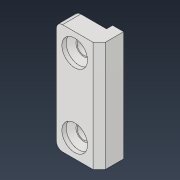
# Autodesk Inventor part: IR Schutz
Saved by Autodesk Inventor 2022.1 (Build 261234020, 234B)
## iProperties
Part Number: IR Schutz
Material: PC/ABS-Kunststoff
Document SubType Name: Modeling
Designer: rYan
Density: 0.357273 g/cm^3
Appearance: Glatt - weiß
Mass: 0.102481 g
Surface Area: 4.81339 cm^2
Volume: 0.286842 cm^3
Author: rYan
Autodesk Inventor part; units mm, degrees
ref_plane "YZ Plane" through (0, 0, 0) normal (1, 0, 0) x (0, 1, 0)
ref_plane "XZ Plane" through (0, 0, 0) normal (0, 1, 0) x (-1, 0, 0)
ref_plane "XY Plane" through (0, 0, 0) normal (0, 0, 1) x (1, 0, 0)
sketch "Skizze1" plane through (0, 0, 0) normal (0, 1, 0) x (-1, 0, 0)
  line L0 (3.5, -9) -> (-3.5, -9)
  line L1 (-3.5, -9) -> (-3.5, 9)
  line L2 (-3.5, 9) -> (3.5, 9)
  line L3 (3.5, 9) -> (3.5, -9)
  line L4 (3.5, -9) -> (-3.5, 9) construction
  line L5 (-3.5, -9) -> (3.5, 9) construction
  line L6 (0.5, 6) -> (0.5, -6) construction
  circle A0 centre (0.5, 6) radius 1.1
  circle A1 centre (0.5, -6) radius 1.1
  point P0 (0, 0)
  dimension "d0" = 7
  dimension "d1" = 18
  dimension "d2" = 2.2
  dimension "d4" = 12
  dimension "d5" = 3
  dimension "d6" = 4
  constraints: 14 end point, 2 centre point, 2 coincident, 2 midpoint, 2 parallel, 1 equal radius, 1 horizontal, 1 perpendicular, 1 vertical
  measures "d0" distance of L1.end L2.end
  measures "d1" distance of L0.end L1.end
  measures "d2" diameter of A0
  measures "d4" distance of L6.start L6.end
  measures "d5" distance from line of L0 L6.end
  measures "d6" distance from line of L1 L6.end
extrude "Extrusion1" add sketch "Skizze1" along normal blind 4
sketch "Skizze3" plane through (0, 4, 0) normal (0, 1, 0) x (1, 0, 0)
  circle A0 centre (-0.5, 6) radius 1.1 projected
  circle A1 centre (-0.5, -6) radius 1.1 projected
  line L0 (3.5, 9) -> (-3.5, 9) projected
  line L1 (-3.5, 9) -> (-3.5, -9) projected
  line L2 (-3.5, -9) -> (3.5, -9) projected
  line L3 (3.5, -9) -> (3.5, 9) projected
  line L4 (1.7, -9) -> (-3.5, -9)
  line L5 (-3.5, -9) -> (-3.5, 9)
  line L6 (-3.5, 9) -> (1.7, 9)
  line L7 (1.7, 9) -> (1.7, -9)
  line L8 (-3.5, -9) -> (3.5, -9) projected
  line L9 (-3.5, 9) -> (-3.5, -9) projected
  line L10 (3.5, 9) -> (-3.5, 9) projected
  point P0 (0, 0)
  dimension "d20" = 1.8
  constraints: 8 end point, 3 collinear
  measures "d20" distance between parallel lines of L3 L7
extrude "Extrusion3" cut sketch "Skizze3" against normal blind 1 contours L7 L2 L1 L0
sketch "Skizze5" plane through (0, 3, 0) normal (0, 1, 0) x (1, 0, 0)
  circle A0 centre (-0.5, -6) radius 1.1 projected
  circle A1 centre (-0.5, 6) radius 1.1 projected
  line L0 (1.7, -9) -> (-3.5, -9) projected
  line L1 (1.7, 9) -> (1.7, -9) projected
  line L2 (-3.5, -9) -> (-3.5, 9) projected
  line L3 (1.7, -4) -> (-0.7, -4)
  line L4 (-0.7, -4) -> (-0.7, 4)
  line L5 (-0.7, 4) -> (1.7, 4)
  line L6 (1.7, 4) -> (1.7, -4)
  line L7 (4.9, 0) -> (-4.9, 0) projected
  line L8 (-3.5, 9) -> (1.7, 9) projected
  point P0 (0, 0)
  dimension "d24" = 8
  dimension "d25" = 2.4
  constraints: 8 end point, 2 parallel, 1 horizontal, 1 perpendicular, 1 point on line, 1 other
  measures "d24" distance of L3.end L4.end
  measures "d25" distance of L3.start L3.end
extrude "Extrusion5" cut sketch "Skizze5" against normal blind 2 contours L3 L4 L7 L1 | L7 L4 L5 L1
sketch "Skizze6" plane through (0, 3, 0) normal (0, 1, 0) x (1, 0, 0)
  line L0 (1.7, -4) -> (-0.7, -4) projected
  line L1 (-0.7, -4) -> (-0.7, 4) projected
  line L2 (-0.7, 4) -> (1.7, 4) projected
  line L3 (1.7, 9) -> (1.7, 4) projected
  line L4 (-3.5, -9) -> (-3.5, 9) projected
  line L5 (1.7, -9) -> (-3.5, -9) projected
  line L6 (1.7, -4) -> (1.7, -9) projected
  circle A0 centre (-0.5, 6) radius 1.1 projected
  circle A1 centre (-0.5, -6) radius 1.1 projected
  line L7 (-0.7, -4) -> (-1.6, -4)
  line L8 (-1.6, 4) -> (-0.7, 4)
  line L9 (-0.7, 4) -> (-0.7, -4)
  line L10 (-1.6, -4.9) -> (-3.5, -4.9)
  line L11 (-3.5, -4.9) -> (-3.5, 4.9)
  line L12 (-3.5, 4.9) -> (-1.6, 4.9)
  line L13 (-1.6, 4.9) -> (-1.6, 4)
  line L14 (-1.6, -4) -> (-1.6, -4.9)
  line L15 (-3.5, 9) -> (1.7, 9) projected
  point P0 (0, 0)
  constraints: 16 end point, 4 parallel, 4 tangent, 2 horizontal, 1 collinear, 1 perpendicular, 1 point on line
extrude "Extrusion6" cut sketch "Skizze6" against normal blind 1.2 contours L7 L14 L10 L4 L12 L13 L8 L1
fillet "Rundung1" radius 1 10 edges at (-3.5, 1.5, 9) (-3.5, 1.5, -9) (-1.6, 2.4, -4.9) (-1.6, 2.4, -4) (-1.6, 2.4, 4) (-1.6, 2.4, 4.9) (1.7, 2, 4) (1.7, 2, -4) (-0.7, 1.4, -4) (-0.7, 1.4, 4)
fillet "Rundung2" radius 0.2 8 edges at (1.4071, 1, 3.7071) (0.5, 1, 4) (-0.4071, 1, 3.7071) (-0.7, 1, 0) (-0.4071, 1, -3.7071) (0.5, 1, -4) (1.4071, 1, -3.7071) (1.7, 1, 0)
chamfer "Fase1" distance 1 angle 45 1 edges at (3.5, 0, 0)
sketch "Skizze7" plane through (0, 0, 0) normal (0, -1, 0) x (1, 0, 0)
  circle A0 centre (-0.5, 6) radius 1.1 projected
  circle A1 centre (-0.5, -6) radius 1.1 projected
  point P0 (0, 0)
  constraints: 2 coincident
hole "Bohrung1" at (-0.5, 0, 6) at (-0.5, 0, -6) direction (0, 1, 0) diameter 4.2 depth 1.5
chamfer "Fase2" distance 0.8 angle 45 2 edges at (-0.5, 1.5, 8.1) (-0.5, 1.5, -3.9)
